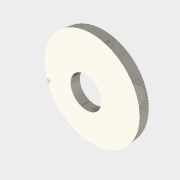
# Autodesk Inventor part: PWTR-0113
Saved by Autodesk Inventor 2021.1 (Build 251245000, 245)
## iProperties
Shininess: 64.0
Length Units: 11269
Angle Units: 11279
Time Units: 11290
Mass Units: 11283
Length Display Precision: 3
Angle Display Precision: 2
Compacted: True
Part Number: PWTR-0113
Document SubType Name: Modeling
Created: 2003-02-05
Designer: B. BOGAN
Material: Stainless Steel, 303
Description: Arm Pivot Pin Washer
Mass: 297.38 g
Surface Area: 177.539 cm^2
Volume: 38.3717 cm^3
Density: 7.75 g/cm^3
Appearance: Titanium - Polished
Vendor: Non-Design Specific
Density: 0.0
Volumn: 0.0
Area: 0.0
PropertySet Name: Model Information
Control State: 0
Master: False
Checked Out: False
Title: PITCH PLATE
Author: B. BOGAN
Revision Number: B
Autodesk Inventor part; units mm, degrees
ref_plane "YZ Plane" through (0, 0, 0) normal (1, 0, 0) x (0, 1, 0)
ref_plane "XZ Plane" through (0, 0, 0) normal (0, 1, 0) x (-1, 0, 0)
ref_plane "XY Plane" through (0, 0, 0) normal (0, 0, 1) x (1, 0, 0)
sketch "Sketch1" plane through (0, 0, 0) normal (0, 0, 1) x (1, 0, 0)
  circle A0 centre (0, 0) radius 15
  dimension "d0" = 30
  constraints: 1 centre point
  measures "d0" diameter of A0
extrude "Extrusion1" add sketch "Sketch1" along normal blind 3
sketch "Sketch2" plane through (0, 0, 3) normal (0, 0, 1) x (1, 0, 0)
  circle A0 centre (0, 0) radius 15 projected
hole "Hole1" at (0, 0, 3) direction (0, 0, -1) diameter 10 end through all
body "Solid1"
